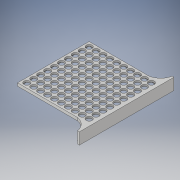
# Autodesk Inventor part: grid
Saved by Autodesk Inventor 2019 (Build 230136000, 136)
## iProperties
Created: 2019-08-01
Part Number: grid
Material: Generic
Document SubType Name: Modeling
Designer: assman
Density: 1 g/cm^3
Appearance: Default
Author: assman
Autodesk Inventor part; units mm, degrees
ref_plane "YZ Plane" through (0, 0, 0) normal (1, 0, 0) x (0, 1, 0)
ref_plane "XZ Plane" through (0, 0, 0) normal (0, 1, 0) x (-1, 0, 0)
ref_plane "XY Plane" through (0, 0, 0) normal (0, 0, 1) x (1, 0, 0)
sketch "Sketch1" plane through (0, 0, 0) normal (0, 1, 0) x (-1, 0, 0)
  line L0 (60.1, 60.1) -> (-60.1, 60.1)
  line L1 (-60.1, 60.1) -> (-60.1, -60.1)
  line L2 (-60.1, -60.1) -> (60.1, -60.1)
  line L3 (60.1, -60.1) -> (60.1, 60.1)
  line L4 (60.1, 60.1) -> (-60.1, -60.1) construction
  line L5 (-60.1, 60.1) -> (60.1, -60.1) construction
  circle A0 centre (-54, 54) radius 5.1
  circle A1 centre (-54, 42) radius 5.1
  circle A2 centre (-54, 30) radius 5.1
  circle A3 centre (-54, 18) radius 5.1
  circle A4 centre (-54, 6) radius 5.1
  circle A5 centre (-54, -6) radius 5.1
  circle A6 centre (-54, -18) radius 5.1
  circle A7 centre (-54, -30) radius 5.1
  circle A8 centre (-54, -42) radius 5.1
  circle A9 centre (-54, -54) radius 5.1
  circle A10 centre (-42, 54) radius 5.1
  circle A11 centre (-42, 42) radius 5.1
  circle A12 centre (-42, 30) radius 5.1
  circle A13 centre (-42, 18) radius 5.1
  circle A14 centre (-42, 6) radius 5.1
  circle A15 centre (-42, -6) radius 5.1
  circle A16 centre (-42, -18) radius 5.1
  circle A17 centre (-42, -30) radius 5.1
  circle A18 centre (-42, -42) radius 5.1
  circle A19 centre (-42, -54) radius 5.1
  circle A20 centre (-30, 54) radius 5.1
  circle A21 centre (-30, 42) radius 5.1
  circle A22 centre (-30, 30) radius 5.1
  circle A23 centre (-30, 18) radius 5.1
  circle A24 centre (-30, 6) radius 5.1
  circle A25 centre (-30, -6) radius 5.1
  circle A26 centre (-30, -18) radius 5.1
  circle A27 centre (-30, -30) radius 5.1
  circle A28 centre (-30, -42) radius 5.1
  circle A29 centre (-30, -54) radius 5.1
  circle A30 centre (-18, 54) radius 5.1
  circle A31 centre (-18, 42) radius 5.1
  circle A32 centre (-18, 30) radius 5.1
  circle A33 centre (-18, 18) radius 5.1
  circle A34 centre (-18, 6) radius 5.1
  circle A35 centre (-18, -6) radius 5.1
  circle A36 centre (-18, -18) radius 5.1
  circle A37 centre (-18, -30) radius 5.1
  circle A38 centre (-18, -42) radius 5.1
  circle A39 centre (-18, -54) radius 5.1
  circle A40 centre (-6, 54) radius 5.1
  circle A41 centre (-6, 42) radius 5.1
  circle A42 centre (-6, 30) radius 5.1
  circle A43 centre (-6, 18) radius 5.1
  circle A44 centre (-6, 6) radius 5.1
  circle A45 centre (-6, -6) radius 5.1
  circle A46 centre (-6, -18) radius 5.1
  circle A47 centre (-6, -30) radius 5.1
  circle A48 centre (-6, -42) radius 5.1
  circle A49 centre (-6, -54) radius 5.1
  circle A50 centre (6, 54) radius 5.1
  circle A51 centre (6, 42) radius 5.1
  circle A52 centre (6, 30) radius 5.1
  circle A53 centre (6, 18) radius 5.1
  circle A54 centre (6, 6) radius 5.1
  circle A55 centre (6, -6) radius 5.1
  circle A56 centre (6, -18) radius 5.1
  circle A57 centre (6, -30) radius 5.1
  circle A58 centre (6, -42) radius 5.1
  circle A59 centre (6, -54) radius 5.1
  circle A60 centre (18, 54) radius 5.1
  circle A61 centre (18, 42) radius 5.1
  circle A62 centre (18, 30) radius 5.1
  circle A63 centre (18, 18) radius 5.1
  circle A64 centre (18, 6) radius 5.1
  circle A65 centre (18, -6) radius 5.1
  circle A66 centre (18, -18) radius 5.1
  circle A67 centre (18, -30) radius 5.1
  circle A68 centre (18, -42) radius 5.1
  circle A69 centre (18, -54) radius 5.1
  circle A70 centre (30, 54) radius 5.1
  circle A71 centre (30, 42) radius 5.1
  circle A72 centre (30, 30) radius 5.1
  circle A73 centre (30, 18) radius 5.1
  circle A74 centre (30, 6) radius 5.1
  circle A75 centre (30, -6) radius 5.1
  circle A76 centre (30, -18) radius 5.1
  circle A77 centre (30, -30) radius 5.1
  circle A78 centre (30, -42) radius 5.1
  circle A79 centre (30, -54) radius 5.1
  circle A80 centre (42, 54) radius 5.1
  circle A81 centre (42, 42) radius 5.1
  circle A82 centre (42, 30) radius 5.1
  circle A83 centre (42, 18) radius 5.1
  circle A84 centre (42, 6) radius 5.1
  circle A85 centre (42, -6) radius 5.1
  circle A86 centre (42, -18) radius 5.1
  circle A87 centre (42, -30) radius 5.1
  circle A88 centre (42, -42) radius 5.1
  circle A89 centre (42, -54) radius 5.1
  circle A90 centre (54, 54) radius 5.1
  circle A91 centre (54, 42) radius 5.1
  circle A92 centre (54, 30) radius 5.1
  circle A93 centre (54, 18) radius 5.1
  circle A94 centre (54, 6) radius 5.1
  circle A95 centre (54, -6) radius 5.1
  circle A96 centre (54, -18) radius 5.1
  circle A97 centre (54, -30) radius 5.1
  circle A98 centre (54, -42) radius 5.1
  circle A99 centre (54, -54) radius 5.1
  point P0 (0, 0)
  dimension "d0" = 120.2
  dimension "d1" = 120.2
  dimension "d2" = 10.2
  dimension "d3" = 6.1
  dimension "d4" = 6.1
  dimension "d7" = 12
  dimension "d10" = 12
  constraints: 100 centre point, 12 end point, 2 horizontal, 2 midpoint, 2 parallel, 1 perpendicular, 1 point on line, 1 vertical, 198 other
  measures "d0" distance of L2.end L1.end
  measures "d1" distance of L1.end L0.end
  measures "d2" diameter of A0
  measures "d3" distance from line of L0 A0.centre
  measures "d4" distance from line of L1 A0.centre
  measures "d7" distance of A0.centre A1.centre
  measures "d10" distance of A0.centre A10.centre
extrude "Extrusion1" add sketch "Sketch1" along normal blind 3
sketch "Sketch2" plane through (0, 3, 0) normal (0, 1, 0) x (1, 0, 0)
  line L0 (60.1, -60.1) -> (60.1, 60.1) projected
  line L1 (-60.1, 60.1) -> (-60.1, -60.1) projected
  line L2 (-60.1, -60.1) -> (60.1, -60.1) projected
  line L3 (60.1, 60.1) -> (-60.1, 60.1) projected
  line L4 (-62.1, -62.1) -> (-62.1, 62.1)
  line L5 (-62.1, 62.1) -> (62.1, 62.1)
  line L6 (62.1, 62.1) -> (62.1, -62.1)
  line L7 (62.1, -62.1) -> (-62.1, -62.1)
  point P0 (0, 0)
  dimension "d17" = 2
  constraints: 8 end point, 3 other
  measures "d17" distance between parallel lines of L1 L4
extrude "Extrusion2" add sketch "Sketch2" against normal blind 5
sketch "Sketch3" plane through (0, 3, 0) normal (0, 1, 0) x (1, 0, 0)
  line L0 (62.1, 62.1) -> (62.1, -62.1) projected
  line L1 (62.1, -62.1) -> (62.1, -82.1)
  line L2 (62.1, 62.1) -> (62.1, -62.1) projected
  line L3 (62.1, 62.1) -> (62.1, 82.1)
  line L4 (62.1, 82.1) -> (65.1, 82.1)
  line L5 (65.1, 82.1) -> (65.1, -82.1)
  line L6 (65.1, -82.1) -> (62.1, -82.1)
  line L7 (62.1, -62.1) -> (-62.1, -62.1) projected
  line L8 (62.1, -62.1) -> (42.1, -62.1)
  line L9 (62.1, 62.1) -> (42.1, 62.1)
  line L10 (-62.1, 62.1) -> (62.1, 62.1) projected
  arc A0 (62.1, -82.1) -> (42.1, -62.1) centre (37.5226, -86.6774) ccw
  arc A1 (42.1, 62.1) -> (62.1, 82.1) centre (37.5226, 86.6774) ccw
  point P0 (0, 0)
  dimension "d20" = 20
  dimension "d21" = 20
  dimension "d22" = 3
  dimension "d23" = 20
  dimension "d24" = 20
  dimension "d25" = 25
  dimension "d26" = 25
  constraints: 14 end point, 4 point on circle, 3 perpendicular, 3 point on line, 2 centre point, 1 vertical
  measures "d20" distance of L0.end L1.end
  measures "d21" distance of L0.start L3.end
  measures "d22" distance of L3.end L4.end
  measures "d23" distance of L0.end L8.end
  measures "d24" distance of L0.start L9.end
  measures "d25" radius of A0
  measures "d26" radius of A1
extrude "Extrusion3" add sketch "Sketch3" against normal blind 20
sketch "Sketch4" plane through (0, -17, 0) normal (0, -1, 0) x (1, 0, 0)
  arc A0 (62.1, -82.1) -> (42.1, -62.1) centre (37.5226, -86.6774) ccw projected
  line L0 (62.1, -62.1) -> (42.1, -62.1) projected
  arc A1 (42.1, 62.1) -> (62.1, 82.1) centre (37.5226, 86.6774) ccw projected
  line L1 (42.1, 62.1) -> (62.1, 62.1) projected
  line L2 (62.1, -82.1) -> (62.1, -62.1)
  line L3 (65.1, -82.1) -> (65.1, 82.1) projected
  line L4 (62.1, -62.1) -> (62.1, 62.1) projected
  line L5 (62.1, 62.1) -> (62.1, 82.1)
  point P0 (0, 0)
  constraints: 4 end point, 1 collinear, 1 parallel
extrude "Extrusion4" cut sketch "Sketch4" against normal blind 15
fillet "Fillet1" radius 10 1 edges at (62.1, -2, 0)
fillet "Fillet2" radius 1 1 edges at (62.1, -17, 0)
body "Solid1"
